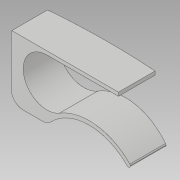
# Autodesk Inventor part: receiving_clip
Saved by Autodesk Inventor 2019.3 (Build 233278000, 278)
## iProperties
Created: 2019-03-03
Part Number: receiving_clip
Material: Generic
Document SubType Name: Modeling
Designer: WW
Density: 1 g/cm^3
Appearance: Default
Author: WW
Autodesk Inventor part; units mm, degrees
ref_plane "YZ Plane" through (0, 0, 0) normal (1, 0, 0) x (0, 1, 0)
ref_plane "XZ Plane" through (0, 0, 0) normal (0, 1, 0) x (-1, 0, 0)
ref_plane "XY Plane" through (0, 0, 0) normal (0, 0, 1) x (1, 0, 0)
sketch "Sketch1" plane through (0, 0, 0) normal (0, 1, 0) x (-1, 0, 0)
  arc A0 (-10, 0) -> (10, 0) centre (0, 113.8115) ccw
  line L0 (10, 0) -> (-10, 0) construction
  line L1 (10, 0) -> (-10, 0)
  line L2 (-10, 0) -> (-10, 6)
  line L3 (-10, 6) -> (10, 6)
  line L4 (10, 6) -> (10, 0)
  point P0 (0, 0)
  point P1 (0, 0)
  dimension "d0" = 114.25
  dimension "d1" = 20
  dimension "d2" = 6
  constraints: 10 end point, 2 horizontal, 2 parallel, 2 point on circle, 1 centre point, 1 coincident, 1 midpoint, 1 perpendicular, 1 vertical alignment
  measures "d0" radius of A0
  measures "d1" distance of L0.end L0.start
  measures "d2" distance of L0.end L2.end
extrude "Extrusion1" add sketch "Sketch1" along normal blind 12
sketch "Sketch2" plane through (-10, 0, 6) normal (0, 0, 1) x (1, 0, 0)
  line L0 (20, 0) -> (0, 0) construction
  line L1 (20, 0) -> (20, 12) construction
  line L2 (0, 12) -> (20, 12) construction
  line L3 (0, 0) -> (0, 12) construction
  circle A0 centre (6, 6) radius 4
  arc A1 (20, 1) -> (8.0951, 2.5925) centre (13.0714, -5.501) ccw
  line L4 (10, 6) -> (10, 0) construction
  line L5 (6, 10) -> (20, 10)
  line L6 (20, 1) -> (20, 0)
  line L7 (20, 0) -> (0, 0) construction
  line L8 (20, 0) -> (0, 0)
  line L9 (0, 0) -> (0, 12)
  line L10 (20, 12) -> (0, 12) construction
  line L11 (20, 12) -> (20, 10)
  line L12 (20, 12) -> (0, 12)
  line L13 (10.6891, 4) -> (16.5284, 4) construction
  arc A2 (20, 0) -> (6.1427, 0) centre (13.0714, -5.501) ccw
  line L14 (20, 1) -> (20, 10)
  point P0 (20, 6)
  dimension "d5" = 8
  dimension "d7" = 1
  dimension "d8" = 2
  dimension "d14" = 2
  constraints: 18 end point, 7 point on circle, 4 tangent, 3 centre point, 3 collinear, 3 point on line, 3 vertical, 2 perpendicular, 1 concentric, 1 horizontal, 1 horizontal alignment, 1 midpoint
  measures "d5" diameter of A0
  measures "d7" distance from line of L0 L6.start
  measures "d8" distance centre to line of A0 L13
  measures "d14" distance between parallel lines of L10 L5
extrude "Extrusion2" cut sketch "Sketch2" against normal through all contours A0 | A0 L5 L14 A1 | L8 A2
fillet "Fillet1" radius 0.32 2 edges at (10, 0, 3) (10, 1, 3)
fillet "Fillet2" radius 2 4 edges at (-3.8573, 0, 2.8133) (-10, 12, 3) (-10, 0, 3) (10, 10, 3)
sketch "Sketch3" plane through (-8, 0, 6) normal (0, 0, 1) x (1, 0, 0)
  arc A0 (16, 10) -> (18, 12) centre (16, 12) ccw construction
  line L0 (0, 12) -> (18, 12) construction
  arc A1 (0, 12) -> (-2, 10) centre (0, 10) ccw construction
  line L1 (-2, 2) -> (-2, 10) construction
  arc A2 (-2, 2) -> (0, 0) centre (0, 2) ccw construction
  line L2 (3.2362, 0) -> (0, 0) construction
  arc A3 (3.2362, 0) -> (4.6809, 0.6169) centre (3.2362, 2) ccw construction
  arc A4 (17.4493, 0.63) -> (4.6809, 0.6169) centre (11.0714, -5.501) ccw construction
  arc A5 (17.4493, 0.63) -> (18, 0.8517) centre (17.68, 0.8517) ccw construction
  line L3 (18, 0.8517) -> (18, 0.8721) construction
  arc A6 (18, 0.8721) -> (17.9103, 1.0943) centre (17.68, 0.8721) ccw construction
  arc A7 (17.9103, 1.0943) -> (6.0951, 2.5925) centre (11.0714, -5.501) ccw construction
  arc A8 (4, 10) -> (6.0951, 2.5925) centre (4, 6) ccw construction
  line L4 (4, 10) -> (16, 10) construction
  line L5 (-2, 12) -> (18, 12)
  line L6 (18, 12) -> (18, 10.6)
  line L7 (18, 10.6) -> (-2, 10.6)
  line L8 (-2, 10.6) -> (-2, 12)
  line L9 (16, 10.6) -> (18, 10.6)
  line L10 (18, 10.6) -> (18, 10)
  line L11 (18, 10) -> (16, 10)
  line L12 (16, 10) -> (16, 10.6)
  point P0 (8, 0)
  dimension "d15" = 20
  dimension "d16" = 1.4
  constraints: 16 end point, 4 parallel, 2 horizontal, 2 perpendicular, 1 point on line
  measures "d15" distance of L6.end L7.end
  measures "d16" distance of L5.end L6.end
extrude "Extrusion3" cut sketch "Sketch3" against normal blind 10
body "Solid1"
